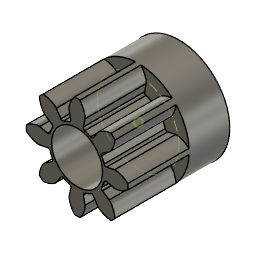
Spur_Gear_Pot (Autodesk Fusion 360 design; units mm, degrees)
description: Spur Gear; Diametrial Pitch: 20.0; Num Teeth: 8; Pressure Angle: 20.0; Backlash: 0.00 in
Autodesk Fusion 360 part; units mm, degrees
(part 1 of 2)
sketch "Sketch1" plane through (0, 0, 7.62) normal (0, 0, 1) x (1, 0, 0)
  arc A0 (5.8346, -2.5905) -> (6.243, -1.3337) centre (0, 0) ccw
  arc A1 (6.5346, -1.1365) -> (6.243, -1.3337) centre (6.4914, -1.3868) ccw
  line L0 (6.5346, -1.1365) -> (7.8387, -1.3616)
  spline S0 degree 5 poles (7.8387, -1.3616) (7.8451, -1.3627) (7.8581, -1.3647) (7.8776, -1.3671) (7.9036, -1.3689) (7.9364, -1.3696) (7.9694, -1.369) (8.0024, -1.3676) (8.0355, -1.3658) (8.0687, -1.3637) (8.1019, -1.3613) (8.1351, -1.3585) (8.1684, -1.3551) (8.2017, -1.3512) (8.235, -1.3466) (8.2684, -1.3414) (8.3019, -1.3357) (8.3353, -1.3297) (8.3688, -1.3232) (8.4023, -1.3164) (8.4358, -1.3093) (8.4693, -1.3017) (8.5028, -1.2938) (8.5363, -1.2855) (8.5698, -1.2768) (8.6034, -1.2677) (8.6369, -1.2583) (8.6704, -1.2484) (8.7039, -1.2383) (8.7374, -1.2278) (8.7709, -1.217) (8.8044, -1.2059) (8.8379, -1.1944) (8.8714, -1.1827) (8.9048, -1.1705) (8.9382, -1.1581) (8.9716, -1.1454) (9.005, -1.1323) (9.0384, -1.1189) (9.0717, -1.1053) (9.105, -1.0913) (9.1383, -1.077) (9.1716, -1.0625) (9.2048, -1.0476) (9.238, -1.0324) (9.2711, -1.017) (9.3042, -1.0013) (9.3373, -0.9852) (9.3703, -0.9689) (9.4033, -0.9524) (9.4363, -0.9355) (9.4692, -0.9184) (9.502, -0.901) (9.5349, -0.8833) (9.5676, -0.8653) (9.6003, -0.8471) (9.633, -0.8286) (9.6656, -0.8098) (9.6982, -0.7908) (9.7307, -0.7715) (9.7632, -0.752) (9.7956, -0.7322) (9.8279, -0.7121) (9.8602, -0.6918) (9.8924, -0.6712) (9.9246, -0.6503) (9.9567, -0.6292) (9.9887, -0.6079) (10.0207, -0.5863) (10.0525, -0.5645) (10.0844, -0.5424) (10.1098, -0.5245) (10.1288, -0.511) (10.1415, -0.5019) (10.1478, -0.4974) knots 0 0 0 0 0 0 0.01428571 0.02857143 0.04285714 0.05714286 0.07142857 0.08571429 0.1 0.11428571 0.12857143 0.14285714 0.15714286 0.17142857 0.18571429 0.2 0.21428571 0.22857143 0.24285714 0.25714286 0.27142857 0.28571429 0.3 0.31428571 0.32857143 0.34285714 0.35714286 0.37142857 0.38571429 0.4 0.41428571 0.42857143 0.44285714 0.45714286 0.47142857 0.48571429 0.5 0.51428571 0.52857143 0.54285714 0.55714286 0.57142857 0.58571429 0.6 0.61428571 0.62857143 0.64285714 0.65714286 0.67142857 0.68571429 0.7 0.71428571 0.72857143 0.74285714 0.75714286 0.77142857 0.78571429 0.8 0.81428571 0.82857143 0.84285714 0.85714286 0.87142857 0.88571429 0.9 0.91428571 0.92857143 0.94285714 0.95714286 0.97142857 0.98571429 1 1 1 1 1 1
  arc A2 (10.1478, -0.4974) -> (10.1478, 0.4974) centre (0, 0) ccw
  spline S1 degree 5 poles (10.1478, 0.4974) (10.1415, 0.5019) (10.1288, 0.511) (10.1098, 0.5245) (10.0844, 0.5424) (10.0525, 0.5645) (10.0207, 0.5863) (9.9887, 0.6079) (9.9567, 0.6292) (9.9246, 0.6503) (9.8924, 0.6712) (9.8602, 0.6918) (9.8279, 0.7121) (9.7956, 0.7322) (9.7632, 0.752) (9.7307, 0.7715) (9.6982, 0.7908) (9.6656, 0.8098) (9.633, 0.8286) (9.6003, 0.8471) (9.5676, 0.8653) (9.5349, 0.8833) (9.502, 0.901) (9.4692, 0.9184) (9.4363, 0.9355) (9.4033, 0.9524) (9.3703, 0.9689) (9.3373, 0.9852) (9.3042, 1.0013) (9.2711, 1.017) (9.238, 1.0324) (9.2048, 1.0476) (9.1716, 1.0625) (9.1383, 1.077) (9.105, 1.0913) (9.0717, 1.1053) (9.0384, 1.1189) (9.005, 1.1323) (8.9716, 1.1454) (8.9382, 1.1581) (8.9048, 1.1705) (8.8714, 1.1827) (8.8379, 1.1944) (8.8044, 1.2059) (8.7709, 1.217) (8.7374, 1.2278) (8.7039, 1.2383) (8.6704, 1.2484) (8.6369, 1.2583) (8.6034, 1.2677) (8.5698, 1.2768) (8.5363, 1.2855) (8.5028, 1.2938) (8.4693, 1.3017) (8.4358, 1.3093) (8.4023, 1.3164) (8.3688, 1.3232) (8.3353, 1.3297) (8.3019, 1.3357) (8.2684, 1.3414) (8.235, 1.3466) (8.2017, 1.3512) (8.1684, 1.3551) (8.1351, 1.3585) (8.1019, 1.3613) (8.0687, 1.3637) (8.0355, 1.3658) (8.0024, 1.3676) (7.9694, 1.369) (7.9364, 1.3696) (7.9036, 1.3689) (7.8776, 1.3671) (7.8581, 1.3647) (7.8451, 1.3627) (7.8387, 1.3616) knots -1 -1 -1 -1 -1 -1 -0.98571429 -0.97142857 -0.95714286 -0.94285714 -0.92857143 -0.91428571 -0.9 -0.88571429 -0.87142857 -0.85714286 -0.84285714 -0.82857143 -0.81428571 -0.8 -0.78571429 -0.77142857 -0.75714286 -0.74285714 -0.72857143 -0.71428571 -0.7 -0.68571429 -0.67142857 -0.65714286 -0.64285714 -0.62857143 -0.61428571 -0.6 -0.58571429 -0.57142857 -0.55714286 -0.54285714 -0.52857143 -0.51428571 -0.5 -0.48571429 -0.47142857 -0.45714286 -0.44285714 -0.42857143 -0.41428571 -0.4 -0.38571429 -0.37142857 -0.35714286 -0.34285714 -0.32857143 -0.31428571 -0.3 -0.28571429 -0.27142857 -0.25714286 -0.24285714 -0.22857143 -0.21428571 -0.2 -0.18571429 -0.17142857 -0.15714286 -0.14285714 -0.12857143 -0.11428571 -0.1 -0.08571429 -0.07142857 -0.05714286 -0.04285714 -0.02857143 -0.01428571 0 0 0 0 0 0
  line L1 (7.8387, 1.3616) -> (6.5346, 1.1365)
  arc A3 (6.243, 1.3337) -> (6.5346, 1.1365) centre (6.4914, 1.3868) ccw
  arc A4 (6.243, 1.3337) -> (5.8346, 2.5905) centre (0, 0) ccw
  arc A5 (5.9546, 2.9215) -> (5.8346, 2.5905) centre (6.0668, 2.6936) ccw
  line L2 (5.9546, 2.9215) -> (7.142, 3.5059)
  spline S2 degree 5 poles (7.142, 3.5059) (7.1478, 3.5088) (7.1595, 3.5148) (7.1766, 3.5243) (7.1988, 3.5382) (7.2257, 3.5569) (7.252, 3.5768) (7.2779, 3.5973) (7.3037, 3.6182) (7.3293, 3.6394) (7.3547, 3.6608) (7.3799, 3.6826) (7.4049, 3.7049) (7.4295, 3.7277) (7.4538, 3.751) (7.4778, 3.7748) (7.5015, 3.7991) (7.525, 3.8237) (7.5483, 3.8486) (7.5714, 3.8737) (7.5943, 3.8992) (7.6169, 3.925) (7.6394, 3.9511) (7.6616, 3.9775) (7.6836, 4.0043) (7.7054, 4.0313) (7.727, 4.0587) (7.7483, 4.0863) (7.7695, 4.1142) (7.7904, 4.1424) (7.8112, 4.1708) (7.8318, 4.1995) (7.8521, 4.2285) (7.8722, 4.2577) (7.8922, 4.2871) (7.9119, 4.3168) (7.9314, 4.3468) (7.9508, 4.377) (7.9699, 4.4074) (7.9888, 4.4381) (8.0076, 4.4689) (8.0261, 4.5) (8.0444, 4.5314) (8.0626, 4.5629) (8.0805, 4.5947) (8.0983, 4.6266) (8.1158, 4.6588) (8.1331, 4.6912) (8.1503, 4.7238) (8.1672, 4.7566) (8.184, 4.7897) (8.2005, 4.8229) (8.2169, 4.8563) (8.233, 4.8899) (8.249, 4.9236) (8.2648, 4.9576) (8.2803, 4.9918) (8.2957, 5.0261) (8.3108, 5.0607) (8.3258, 5.0954) (8.3406, 5.1303) (8.3551, 5.1654) (8.3695, 5.2006) (8.3837, 5.236) (8.3976, 5.2716) (8.4114, 5.3074) (8.425, 5.3433) (8.4383, 5.3794) (8.4515, 5.4157) (8.4645, 5.4521) (8.4772, 5.4887) (8.4873, 5.518) (8.4947, 5.5402) (8.4997, 5.5549) (8.5021, 5.5623) knots 0 0 0 0 0 0 0.01428571 0.02857143 0.04285714 0.05714286 0.07142857 0.08571429 0.1 0.11428571 0.12857143 0.14285714 0.15714286 0.17142857 0.18571429 0.2 0.21428571 0.22857143 0.24285714 0.25714286 0.27142857 0.28571429 0.3 0.31428571 0.32857143 0.34285714 0.35714286 0.37142857 0.38571429 0.4 0.41428571 0.42857143 0.44285714 0.45714286 0.47142857 0.48571429 0.5 0.51428571 0.52857143 0.54285714 0.55714286 0.57142857 0.58571429 0.6 0.61428571 0.62857143 0.64285714 0.65714286 0.67142857 0.68571429 0.7 0.71428571 0.72857143 0.74285714 0.75714286 0.77142857 0.78571429 0.8 0.81428571 0.82857143 0.84285714 0.85714286 0.87142857 0.88571429 0.9 0.91428571 0.92857143 0.94285714 0.95714286 0.97142857 0.98571429 1 1 1 1 1 1
  arc A6 (8.5021, 5.5623) -> (7.9174, 6.3671) centre (0, 0) ccw
  spline S3 degree 5 poles (7.9174, 6.3671) (7.9096, 6.3671) (7.894, 6.367) (7.8707, 6.3667) (7.8396, 6.3662) (7.8009, 6.3654) (7.7623, 6.3643) (7.7237, 6.363) (7.6852, 6.3615) (7.6469, 6.3596) (7.6086, 6.3576) (7.5705, 6.3553) (7.5324, 6.3528) (7.4944, 6.35) (7.4566, 6.347) (7.4188, 6.3437) (7.3812, 6.3402) (7.3437, 6.3365) (7.3062, 6.3325) (7.2689, 6.3283) (7.2317, 6.3238) (7.1947, 6.319) (7.1577, 6.314) (7.1209, 6.3088) (7.0842, 6.3033) (7.0477, 6.2976) (7.0112, 6.2916) (6.9749, 6.2854) (6.9387, 6.2789) (6.9027, 6.2722) (6.8668, 6.2652) (6.8311, 6.2579) (6.7954, 6.2504) (6.76, 6.2427) (6.7247, 6.2347) (6.6895, 6.2264) (6.6545, 6.2179) (6.6197, 6.2091) (6.585, 6.2) (6.5505, 6.1907) (6.5161, 6.1811) (6.4819, 6.1713) (6.4479, 6.1611) (6.4141, 6.1507) (6.3805, 6.14) (6.347, 6.1291) (6.3138, 6.1179) (6.2807, 6.1064) (6.2478, 6.0946) (6.2151, 6.0825) (6.1827, 6.0702) (6.1504, 6.0575) (6.1184, 6.0445) (6.0866, 6.0313) (6.0551, 6.0176) (6.0238, 6.0037) (5.9927, 5.9896) (5.9619, 5.9751) (5.9312, 5.9604) (5.9009, 5.9453) (5.8708, 5.9298) (5.8411, 5.9139) (5.8118, 5.8976) (5.7829, 5.8807) (5.7544, 5.8635) (5.7261, 5.8459) (5.6981, 5.8281) (5.6702, 5.8101) (5.6427, 5.7918) (5.6157, 5.7729) (5.5895, 5.7531) (5.5695, 5.7363) (5.5552, 5.7229) (5.5459, 5.7137) (5.5413, 5.709) knots -1 -1 -1 -1 -1 -1 -0.98571429 -0.97142857 -0.95714286 -0.94285714 -0.92857143 -0.91428571 -0.9 -0.88571429 -0.87142857 -0.85714286 -0.84285714 -0.82857143 -0.81428571 -0.8 -0.78571429 -0.77142857 -0.75714286 -0.74285714 -0.72857143 -0.71428571 -0.7 -0.68571429 -0.67142857 -0.65714286 -0.64285714 -0.62857143 -0.61428571 -0.6 -0.58571429 -0.57142857 -0.55714286 -0.54285714 -0.52857143 -0.51428571 -0.5 -0.48571429 -0.47142857 -0.45714286 -0.44285714 -0.42857143 -0.41428571 -0.4 -0.38571429 -0.37142857 -0.35714286 -0.34285714 -0.32857143 -0.31428571 -0.3 -0.28571429 -0.27142857 -0.25714286 -0.24285714 -0.22857143 -0.21428571 -0.2 -0.18571429 -0.17142857 -0.15714286 -0.14285714 -0.12857143 -0.11428571 -0.1 -0.08571429 -0.07142857 -0.05714286 -0.04285714 -0.02857143 -0.01428571 0 0 0 0 0 0
  line L3 (5.5413, 5.709) -> (4.6186, 4.7604)
  arc A7 (4.2667, 4.7485) -> (4.6186, 4.7604) centre (4.4365, 4.9375) ccw
  arc A8 (4.2667, 4.7485) -> (3.1976, 5.5253) centre (0, 0) ccw
  arc A9 (3.1002, 5.8636) -> (3.1976, 5.5253) centre (3.3249, 5.7451) ccw
  line L4 (3.1002, 5.8636) -> (3.7172, 7.0343)
  spline S4 degree 5 poles (3.7172, 7.0343) (3.7203, 7.0401) (3.7262, 7.0518) (3.7344, 7.0696) (3.7443, 7.0938) (3.755, 7.1248) (3.7646, 7.1563) (3.7735, 7.1881) (3.7821, 7.2202) (3.7903, 7.2524) (3.7983, 7.2847) (3.8059, 7.3171) (3.813, 7.3498) (3.8195, 7.3827) (3.8254, 7.4159) (3.8308, 7.4492) (3.8358, 7.4828) (3.8403, 7.5165) (3.8446, 7.5503) (3.8484, 7.5843) (3.852, 7.6183) (3.8552, 7.6525) (3.858, 7.6868) (3.8605, 7.7213) (3.8625, 7.7558) (3.8643, 7.7905) (3.8656, 7.8254) (3.8667, 7.8603) (3.8674, 7.8953) (3.8678, 7.9304) (3.8678, 7.9656) (3.8676, 8.0009) (3.8671, 8.0362) (3.8662, 8.0717) (3.865, 8.1073) (3.8635, 8.1429) (3.8617, 8.1786) (3.8596, 8.2144) (3.8572, 8.2502) (3.8545, 8.2862) (3.8515, 8.3222) (3.8482, 8.3582) (3.8446, 8.3943) (3.8407, 8.4305) (3.8366, 8.4668) (3.8321, 8.5031) (3.8274, 8.5394) (3.8224, 8.5758) (3.8171, 8.6123) (3.8115, 8.6488) (3.8057, 8.6853) (3.7996, 8.7219) (3.7932, 8.7586) (3.7865, 8.7952) (3.7795, 8.832) (3.7723, 8.8687) (3.7648, 8.9055) (3.757, 8.9423) (3.749, 8.9792) (3.7407, 9.016) (3.7322, 9.0529) (3.7233, 9.0899) (3.7142, 9.1268) (3.7049, 9.1638) (3.6953, 9.2008) (3.6854, 9.2379) (3.6752, 9.2749) (3.6648, 9.312) (3.6542, 9.349) (3.6433, 9.3861) (3.6321, 9.4232) (3.6229, 9.4529) (3.616, 9.4752) (3.6113, 9.49) (3.6089, 9.4974) knots 0 0 0 0 0 0 0.01428571 0.02857143 0.04285714 0.05714286 0.07142857 0.08571429 0.1 0.11428571 0.12857143 0.14285714 0.15714286 0.17142857 0.18571429 0.2 0.21428571 0.22857143 0.24285714 0.25714286 0.27142857 0.28571429 0.3 0.31428571 0.32857143 0.34285714 0.35714286 0.37142857 0.38571429 0.4 0.41428571 0.42857143 0.44285714 0.45714286 0.47142857 0.48571429 0.5 0.51428571 0.52857143 0.54285714 0.55714286 0.57142857 0.58571429 0.6 0.61428571 0.62857143 0.64285714 0.65714286 0.67142857 0.68571429 0.7 0.71428571 0.72857143 0.74285714 0.75714286 0.77142857 0.78571429 0.8 0.81428571 0.82857143 0.84285714 0.85714286 0.87142857 0.88571429 0.9 0.91428571 0.92857143 0.94285714 0.95714286 0.97142857 0.98571429 1 1 1 1 1 1
  arc A10 (3.6089, 9.4974) -> (2.6628, 9.8049) centre (0, 0) ccw
  spline S5 degree 5 poles (2.6628, 9.8049) (2.6565, 9.8002) (2.644, 9.791) (2.6253, 9.7771) (2.6004, 9.7584) (2.5696, 9.735) (2.5389, 9.7114) (2.5085, 9.6877) (2.4783, 9.6638) (2.4483, 9.6398) (2.4186, 9.6156) (2.3891, 9.5914) (2.3598, 9.5669) (2.3307, 9.5424) (2.3018, 9.5177) (2.2732, 9.4929) (2.2448, 9.4679) (2.2166, 9.4428) (2.1887, 9.4176) (2.161, 9.3922) (2.1336, 9.3667) (2.1064, 9.3411) (2.0794, 9.3154) (2.0527, 9.2895) (2.0262, 9.2635) (2, 9.2374) (1.9741, 9.2111) (1.9484, 9.1847) (1.9229, 9.1582) (1.8977, 9.1316) (1.8728, 9.1049) (1.8481, 9.078) (1.8237, 9.051) (1.7996, 9.0239) (1.7757, 8.9966) (1.7522, 8.9693) (1.7289, 8.9418) (1.7058, 8.9142) (1.6831, 8.8865) (1.6606, 8.8586) (1.6385, 8.8307) (1.6166, 8.8026) (1.5951, 8.7745) (1.5738, 8.7462) (1.5529, 8.7178) (1.5323, 8.6892) (1.512, 8.6606) (1.492, 8.6319) (1.4723, 8.603) (1.4529, 8.574) (1.4339, 8.545) (1.4153, 8.5158) (1.397, 8.4865) (1.3791, 8.457) (1.3616, 8.4275) (1.3445, 8.3978) (1.3276, 8.3681) (1.3112, 8.3383) (1.2951, 8.3083) (1.2793, 8.2783) (1.2641, 8.2481) (1.2494, 8.2178) (1.2353, 8.1873) (1.2219, 8.1567) (1.2089, 8.126) (1.1964, 8.0952) (1.1842, 8.0643) (1.1722, 8.0334) (1.1607, 8.0024) (1.15, 7.9712) (1.1404, 7.9398) (1.1342, 7.9144) (1.1304, 7.8952) (1.1283, 7.8823) (1.1273, 7.8758) knots -1 -1 -1 -1 -1 -1 -0.98571429 -0.97142857 -0.95714286 -0.94285714 -0.92857143 -0.91428571 -0.9 -0.88571429 -0.87142857 -0.85714286 -0.84285714 -0.82857143 -0.81428571 -0.8 -0.78571429 -0.77142857 -0.75714286 -0.74285714 -0.72857143 -0.71428571 -0.7 -0.68571429 -0.67142857 -0.65714286 -0.64285714 -0.62857143 -0.61428571 -0.6 -0.58571429 -0.57142857 -0.55714286 -0.54285714 -0.52857143 -0.51428571 -0.5 -0.48571429 -0.47142857 -0.45714286 -0.44285714 -0.42857143 -0.41428571 -0.4 -0.38571429 -0.37142857 -0.35714286 -0.34285714 -0.32857143 -0.31428571 -0.3 -0.28571429 -0.27142857 -0.25714286 -0.24285714 -0.22857143 -0.21428571 -0.2 -0.18571429 -0.17142857 -0.15714286 -0.14285714 -0.12857143 -0.11428571 -0.1 -0.08571429 -0.07142857 -0.05714286 -0.04285714 -0.02857143 -0.01428571 0 0 0 0 0 0
  line L5 (1.1273, 7.8758) -> (0.9384, 6.566)
  arc A11 (0.6607, 6.3496) -> (0.9384, 6.566) centre (0.687, 6.6022) ccw
  arc A12 (0.6607, 6.3496) -> (-0.6607, 6.3496) centre (0, 0) ccw
  arc A13 (-0.9384, 6.566) -> (-0.6607, 6.3496) centre (-0.687, 6.6022) ccw
  line L6 (-0.9384, 6.566) -> (-1.1273, 7.8758)
  spline S6 degree 5 poles (-1.1273, 7.8758) (-1.1283, 7.8823) (-1.1304, 7.8952) (-1.1342, 7.9144) (-1.1404, 7.9398) (-1.15, 7.9712) (-1.1607, 8.0024) (-1.1722, 8.0334) (-1.1842, 8.0643) (-1.1964, 8.0952) (-1.2089, 8.126) (-1.2219, 8.1567) (-1.2353, 8.1873) (-1.2494, 8.2178) (-1.2641, 8.2481) (-1.2793, 8.2783) (-1.2951, 8.3083) (-1.3112, 8.3383) (-1.3276, 8.3681) (-1.3445, 8.3978) (-1.3616, 8.4275) (-1.3791, 8.457) (-1.397, 8.4865) (-1.4153, 8.5158) (-1.4339, 8.545) (-1.4529, 8.574) (-1.4723, 8.603) (-1.492, 8.6319) (-1.512, 8.6606) (-1.5323, 8.6892) (-1.5529, 8.7178) (-1.5738, 8.7462) (-1.5951, 8.7745) (-1.6166, 8.8026) (-1.6385, 8.8307) (-1.6606, 8.8586) (-1.6831, 8.8865) (-1.7058, 8.9142) (-1.7289, 8.9418) (-1.7522, 8.9693) (-1.7757, 8.9966) (-1.7996, 9.0239) (-1.8237, 9.051) (-1.8481, 9.078) (-1.8728, 9.1049) (-1.8977, 9.1316) (-1.9229, 9.1582) (-1.9484, 9.1847) (-1.9741, 9.2111) (-2, 9.2374) (-2.0262, 9.2635) (-2.0527, 9.2895) (-2.0794, 9.3154) (-2.1064, 9.3411) (-2.1336, 9.3667) (-2.161, 9.3922) (-2.1887, 9.4176) (-2.2166, 9.4428) (-2.2448, 9.4679) (-2.2732, 9.4929) (-2.3018, 9.5177) (-2.3307, 9.5424) (-2.3598, 9.5669) (-2.3891, 9.5914) (-2.4186, 9.6156) (-2.4483, 9.6398) (-2.4783, 9.6638) (-2.5085, 9.6877) (-2.5389, 9.7114) (-2.5696, 9.735) (-2.6004, 9.7584) (-2.6253, 9.7771) (-2.644, 9.791) (-2.6565, 9.8002) (-2.6628, 9.8049) knots 0 0 0 0 0 0 0.01428571 0.02857143 0.04285714 0.05714286 0.07142857 0.08571429 0.1 0.11428571 0.12857143 0.14285714 0.15714286 0.17142857 0.18571429 0.2 0.21428571 0.22857143 0.24285714 0.25714286 0.27142857 0.28571429 0.3 0.31428571 0.32857143 0.34285714 0.35714286 0.37142857 0.38571429 0.4 0.41428571 0.42857143 0.44285714 0.45714286 0.47142857 0.48571429 0.5 0.51428571 0.52857143 0.54285714 0.55714286 0.57142857 0.58571429 0.6 0.61428571 0.62857143 0.64285714 0.65714286 0.67142857 0.68571429 0.7 0.71428571 0.72857143 0.74285714 0.75714286 0.77142857 0.78571429 0.8 0.81428571 0.82857143 0.84285714 0.85714286 0.87142857 0.88571429 0.9 0.91428571 0.92857143 0.94285714 0.95714286 0.97142857 0.98571429 1 1 1 1 1 1
  arc A14 (-2.6628, 9.8049) -> (-3.6089, 9.4974) centre (0, 0) ccw
  spline S7 degree 5 poles (-3.6089, 9.4974) (-3.6113, 9.49) (-3.616, 9.4752) (-3.6229, 9.4529) (-3.6321, 9.4232) (-3.6433, 9.3861) (-3.6542, 9.349) (-3.6648, 9.312) (-3.6752, 9.2749) (-3.6854, 9.2379) (-3.6953, 9.2008) (-3.7049, 9.1638) (-3.7142, 9.1268) (-3.7233, 9.0899) (-3.7322, 9.0529) (-3.7407, 9.016) (-3.749, 8.9792) (-3.757, 8.9423) (-3.7648, 8.9055) (-3.7723, 8.8687) (-3.7795, 8.832) (-3.7865, 8.7952) (-3.7932, 8.7586) (-3.7996, 8.7219) (-3.8057, 8.6853) (-3.8115, 8.6488) (-3.8171, 8.6123) (-3.8224, 8.5758) (-3.8274, 8.5394) (-3.8321, 8.5031) (-3.8366, 8.4668) (-3.8407, 8.4305) (-3.8446, 8.3943) (-3.8482, 8.3582) (-3.8515, 8.3222) (-3.8545, 8.2862) (-3.8572, 8.2502) (-3.8596, 8.2144) (-3.8617, 8.1786) (-3.8635, 8.1429) (-3.865, 8.1073) (-3.8662, 8.0717) (-3.8671, 8.0362) (-3.8676, 8.0009) (-3.8678, 7.9656) (-3.8678, 7.9304) (-3.8674, 7.8953) (-3.8667, 7.8603) (-3.8656, 7.8254) (-3.8643, 7.7905) (-3.8625, 7.7558) (-3.8605, 7.7213) (-3.858, 7.6868) (-3.8552, 7.6525) (-3.852, 7.6183) (-3.8484, 7.5843) (-3.8446, 7.5503) (-3.8403, 7.5165) (-3.8358, 7.4828) (-3.8308, 7.4492) (-3.8254, 7.4159) (-3.8195, 7.3827) (-3.813, 7.3498) (-3.8059, 7.3171) (-3.7983, 7.2847) (-3.7903, 7.2524) (-3.7821, 7.2202) (-3.7735, 7.1881) (-3.7646, 7.1563) (-3.755, 7.1248) (-3.7443, 7.0938) (-3.7344, 7.0696) (-3.7262, 7.0518) (-3.7203, 7.0401) (-3.7172, 7.0343) knots -1 -1 -1 -1 -1 -1 -0.98571429 -0.97142857 -0.95714286 -0.94285714 -0.92857143 -0.91428571 -0.9 -0.88571429 -0.87142857 -0.85714286 -0.84285714 -0.82857143 -0.81428571 -0.8 -0.78571429 -0.77142857 -0.75714286 -0.74285714 -0.72857143 -0.71428571 -0.7 -0.68571429 -0.67142857 -0.65714286 -0.64285714 -0.62857143 -0.61428571 -0.6 -0.58571429 -0.57142857 -0.55714286 -0.54285714 -0.52857143 -0.51428571 -0.5 -0.48571429 -0.47142857 -0.45714286 -0.44285714 -0.42857143 -0.41428571 -0.4 -0.38571429 -0.37142857 -0.35714286 -0.34285714 -0.32857143 -0.31428571 -0.3 -0.28571429 -0.27142857 -0.25714286 -0.24285714 -0.22857143 -0.21428571 -0.2 -0.18571429 -0.17142857 -0.15714286 -0.14285714 -0.12857143 -0.11428571 -0.1 -0.08571429 -0.07142857 -0.05714286 -0.04285714 -0.02857143 -0.01428571 0 0 0 0 0 0
  line L7 (-3.7172, 7.0343) -> (-3.1002, 5.8636)
  arc A15 (-3.1976, 5.5253) -> (-3.1002, 5.8636) centre (-3.3249, 5.7451) ccw
  arc A16 (-3.1976, 5.5253) -> (-4.2667, 4.7485) centre (0, 0) ccw
  arc A17 (-4.6186, 4.7604) -> (-4.2667, 4.7485) centre (-4.4365, 4.9375) ccw
  line L8 (-4.6186, 4.7604) -> (-5.5413, 5.709)
  spline S8 degree 5 poles (-5.5413, 5.709) (-5.5459, 5.7137) (-5.5552, 5.7229) (-5.5695, 5.7363) (-5.5895, 5.7531) (-5.6157, 5.7729) (-5.6427, 5.7918) (-5.6702, 5.8101) (-5.6981, 5.8281) (-5.7261, 5.8459) (-5.7544, 5.8635) (-5.7829, 5.8807) (-5.8118, 5.8976) (-5.8411, 5.9139) (-5.8708, 5.9298) (-5.9009, 5.9453) (-5.9312, 5.9604) (-5.9619, 5.9751) (-5.9927, 5.9896) (-6.0238, 6.0037) (-6.0551, 6.0176) (-6.0866, 6.0313) (-6.1184, 6.0445) (-6.1504, 6.0575) (-6.1827, 6.0702) (-6.2151, 6.0825) (-6.2478, 6.0946) (-6.2807, 6.1064) (-6.3138, 6.1179) (-6.347, 6.1291) (-6.3805, 6.14) (-6.4141, 6.1507) (-6.4479, 6.1611) (-6.4819, 6.1713) (-6.5161, 6.1811) (-6.5505, 6.1907) (-6.585, 6.2) (-6.6197, 6.2091) (-6.6545, 6.2179) (-6.6895, 6.2264) (-6.7247, 6.2347) (-6.76, 6.2427) (-6.7954, 6.2504) (-6.8311, 6.2579) (-6.8668, 6.2652) (-6.9027, 6.2722) (-6.9387, 6.2789) (-6.9749, 6.2854) (-7.0112, 6.2916) (-7.0477, 6.2976) (-7.0842, 6.3033) (-7.1209, 6.3088) (-7.1577, 6.314) (-7.1947, 6.319) (-7.2317, 6.3238) (-7.2689, 6.3283) (-7.3062, 6.3325) (-7.3437, 6.3365) (-7.3812, 6.3402) (-7.4188, 6.3437) (-7.4566, 6.347) (-7.4944, 6.35) (-7.5324, 6.3528) (-7.5705, 6.3553) (-7.6086, 6.3576) (-7.6469, 6.3596) (-7.6852, 6.3615) (-7.7237, 6.363) (-7.7623, 6.3643) (-7.8009, 6.3654) (-7.8396, 6.3662) (-7.8707, 6.3667) (-7.894, 6.367) (-7.9096, 6.3671) (-7.9174, 6.3671) knots 0 0 0 0 0 0 0.01428571 0.02857143 0.04285714 0.05714286 0.07142857 0.08571429 0.1 0.11428571 0.12857143 0.14285714 0.15714286 0.17142857 0.18571429 0.2 0.21428571 0.22857143 0.24285714 0.25714286 0.27142857 0.28571429 0.3 0.31428571 0.32857143 0.34285714 0.35714286 0.37142857 0.38571429 0.4 0.41428571 0.42857143 0.44285714 0.45714286 0.47142857 0.48571429 0.5 0.51428571 0.52857143 0.54285714 0.55714286 0.57142857 0.58571429 0.6 0.61428571 0.62857143 0.64285714 0.65714286 0.67142857 0.68571429 0.7 0.71428571 0.72857143 0.74285714 0.75714286 0.77142857 0.78571429 0.8 0.81428571 0.82857143 0.84285714 0.85714286 0.87142857 0.88571429 0.9 0.91428571 0.92857143 0.94285714 0.95714286 0.97142857 0.98571429 1 1 1 1 1 1
  arc A18 (-7.9174, 6.3671) -> (-8.5021, 5.5623) centre (0, 0) ccw
  spline S9 degree 5 poles (-8.5021, 5.5623) (-8.4997, 5.5549) (-8.4947, 5.5402) (-8.4873, 5.518) (-8.4772, 5.4887) (-8.4645, 5.4521) (-8.4515, 5.4157) (-8.4383, 5.3794) (-8.425, 5.3433) (-8.4114, 5.3074) (-8.3976, 5.2716) (-8.3837, 5.236) (-8.3695, 5.2006) (-8.3551, 5.1654) (-8.3406, 5.1303) (-8.3258, 5.0954) (-8.3108, 5.0607) (-8.2957, 5.0261) (-8.2803, 4.9918) (-8.2648, 4.9576) (-8.249, 4.9236) (-8.233, 4.8899) (-8.2169, 4.8563) (-8.2005, 4.8229) (-8.184, 4.7897) (-8.1672, 4.7566) (-8.1503, 4.7238) (-8.1331, 4.6912) (-8.1158, 4.6588) (-8.0983, 4.6266) (-8.0805, 4.5947) (-8.0626, 4.5629) (-8.0444, 4.5314) (-8.0261, 4.5) (-8.0076, 4.4689) (-7.9888, 4.4381) (-7.9699, 4.4074) (-7.9508, 4.377) (-7.9314, 4.3468) (-7.9119, 4.3168) (-7.8922, 4.2871) (-7.8722, 4.2577) (-7.8521, 4.2285) (-7.8318, 4.1995) (-7.8112, 4.1708) (-7.7904, 4.1424) (-7.7695, 4.1142) (-7.7483, 4.0863) (-7.727, 4.0587) (-7.7054, 4.0313) (-7.6836, 4.0043) (-7.6616, 3.9775) (-7.6394, 3.9511) (-7.6169, 3.925) (-7.5943, 3.8992) (-7.5714, 3.8737) (-7.5483, 3.8486) (-7.525, 3.8237) (-7.5015, 3.7991) (-7.4778, 3.7748) (-7.4538, 3.751) (-7.4295, 3.7277) (-7.4049, 3.7049) (-7.3799, 3.6826) (-7.3547, 3.6608) (-7.3293, 3.6394) (-7.3037, 3.6182) (-7.2779, 3.5973) (-7.252, 3.5768) (-7.2257, 3.5569) (-7.1988, 3.5382) (-7.1766, 3.5243) (-7.1595, 3.5148) (-7.1478, 3.5088) (-7.142, 3.5059) knots -1 -1 -1 -1 -1 -1 -0.98571429 -0.97142857 -0.95714286 -0.94285714 -0.92857143 -0.91428571 -0.9 -0.88571429 -0.87142857 -0.85714286 -0.84285714 -0.82857143 -0.81428571 -0.8 -0.78571429 -0.77142857 -0.75714286 -0.74285714 -0.72857143 -0.71428571 -0.7 -0.68571429 -0.67142857 -0.65714286 -0.64285714 -0.62857143 -0.61428571 -0.6 -0.58571429 -0.57142857 -0.55714286 -0.54285714 -0.52857143 -0.51428571 -0.5 -0.48571429 -0.47142857 -0.45714286 -0.44285714 -0.42857143 -0.41428571 -0.4 -0.38571429 -0.37142857 -0.35714286 -0.34285714 -0.32857143 -0.31428571 -0.3 -0.28571429 -0.27142857 -0.25714286 -0.24285714 -0.22857143 -0.21428571 -0.2 -0.18571429 -0.17142857 -0.15714286 -0.14285714 -0.12857143 -0.11428571 -0.1 -0.08571429 -0.07142857 -0.05714286 -0.04285714 -0.02857143 -0.01428571 0 0 0 0 0 0
  line L9 (-7.142, 3.5059) -> (-5.9546, 2.9215)
  arc A19 (-5.8346, 2.5905) -> (-5.9546, 2.9215) centre (-6.0668, 2.6936) ccw
  arc A20 (-5.8346, 2.5905) -> (-6.243, 1.3337) centre (0, 0) ccw
  arc A21 (-6.5346, 1.1365) -> (-6.243, 1.3337) centre (-6.4914, 1.3868) ccw
  line L10 (-6.5346, 1.1365) -> (-7.8387, 1.3616)
  spline S10 degree 5 poles (-7.8387, 1.3616) (-7.8451, 1.3627) (-7.8581, 1.3647) (-7.8776, 1.3671) (-7.9036, 1.3689) (-7.9364, 1.3696) (-7.9694, 1.369) (-8.0024, 1.3676) (-8.0355, 1.3658) (-8.0687, 1.3637) (-8.1019, 1.3613) (-8.1351, 1.3585) (-8.1684, 1.3551) (-8.2017, 1.3512) (-8.235, 1.3466) (-8.2684, 1.3414) (-8.3019, 1.3357) (-8.3353, 1.3297) (-8.3688, 1.3232) (-8.4023, 1.3164) (-8.4358, 1.3093) (-8.4693, 1.3017) (-8.5028, 1.2938) (-8.5363, 1.2855) (-8.5698, 1.2768) (-8.6034, 1.2677) (-8.6369, 1.2583) (-8.6704, 1.2484) (-8.7039, 1.2383) (-8.7374, 1.2278) (-8.7709, 1.217) (-8.8044, 1.2059) (-8.8379, 1.1944) (-8.8714, 1.1827) (-8.9048, 1.1705) (-8.9382, 1.1581) (-8.9716, 1.1454) (-9.005, 1.1323) (-9.0384, 1.1189) (-9.0717, 1.1053) (-9.105, 1.0913) (-9.1383, 1.077) (-9.1716, 1.0625) (-9.2048, 1.0476) (-9.238, 1.0324) (-9.2711, 1.017) (-9.3042, 1.0013) (-9.3373, 0.9852) (-9.3703, 0.9689) (-9.4033, 0.9524) (-9.4363, 0.9355) (-9.4692, 0.9184) (-9.502, 0.901) (-9.5349, 0.8833) (-9.5676, 0.8653) (-9.6003, 0.8471) (-9.633, 0.8286) (-9.6656, 0.8098) (-9.6982, 0.7908) (-9.7307, 0.7715) (-9.7632, 0.752) (-9.7956, 0.7322) (-9.8279, 0.7121) (-9.8602, 0.6918) (-9.8924, 0.6712) (-9.9246, 0.6503) (-9.9567, 0.6292) (-9.9887, 0.6079) (-10.0207, 0.5863) (-10.0525, 0.5645) (-10.0844, 0.5424) (-10.1098, 0.5245) (-10.1288, 0.511) (-10.1415, 0.5019) (-10.1478, 0.4974) knots 0 0 0 0 0 0 0.01428571 0.02857143 0.04285714 0.05714286 0.07142857 0.08571429 0.1 0.11428571 0.12857143 0.14285714 0.15714286 0.17142857 0.18571429 0.2 0.21428571 0.22857143 0.24285714 0.25714286 0.27142857 0.28571429 0.3 0.31428571 0.32857143 0.34285714 0.35714286 0.37142857 0.38571429 0.4 0.41428571 0.42857143 0.44285714 0.45714286 0.47142857 0.48571429 0.5 0.51428571 0.52857143 0.54285714 0.55714286 0.57142857 0.58571429 0.6 0.61428571 0.62857143 0.64285714 0.65714286 0.67142857 0.68571429 0.7 0.71428571 0.72857143 0.74285714 0.75714286 0.77142857 0.78571429 0.8 0.81428571 0.82857143 0.84285714 0.85714286 0.87142857 0.88571429 0.9 0.91428571 0.92857143 0.94285714 0.95714286 0.97142857 0.98571429 1 1 1 1 1 1
  arc A22 (-10.1478, 0.4974) -> (-10.1478, -0.4974) centre (0, 0) ccw
  spline S11 degree 5 poles (-10.1478, -0.4974) (-10.1415, -0.5019) (-10.1288, -0.511) (-10.1098, -0.5245) (-10.0844, -0.5424) (-10.0525, -0.5645) (-10.0207, -0.5863) (-9.9887, -0.6079) (-9.9567, -0.6292) (-9.9246, -0.6503) (-9.8924, -0.6712) (-9.8602, -0.6918) (-9.8279, -0.7121) (-9.7956, -0.7322) (-9.7632, -0.752) (-9.7307, -0.7715) (-9.6982, -0.7908) (-9.6656, -0.8098) (-9.633, -0.8286) (-9.6003, -0.8471) (-9.5676, -0.8653) (-9.5349, -0.8833) (-9.502, -0.901) (-9.4692, -0.9184) (-9.4363, -0.9355) (-9.4033, -0.9524) (-9.3703, -0.9689) (-9.3373, -0.9852) (-9.3042, -1.0013) (-9.2711, -1.017) (-9.238, -1.0324) (-9.2048, -1.0476) (-9.1716, -1.0625) (-9.1383, -1.077) (-9.105, -1.0913) (-9.0717, -1.1053) (-9.0384, -1.1189) (-9.005, -1.1323) (-8.9716, -1.1454) (-8.9382, -1.1581) (-8.9048, -1.1705) (-8.8714, -1.1827) (-8.8379, -1.1944) (-8.8044, -1.2059) (-8.7709, -1.217) (-8.7374, -1.2278) (-8.7039, -1.2383) (-8.6704, -1.2484) (-8.6369, -1.2583) (-8.6034, -1.2677) (-8.5698, -1.2768) (-8.5363, -1.2855) (-8.5028, -1.2938) (-8.4693, -1.3017) (-8.4358, -1.3093) (-8.4023, -1.3164) (-8.3688, -1.3232) (-8.3353, -1.3297) (-8.3019, -1.3357) (-8.2684, -1.3414) (-8.235, -1.3466) (-8.2017, -1.3512) (-8.1684, -1.3551) (-8.1351, -1.3585) (-8.1019, -1.3613) (-8.0687, -1.3637) (-8.0355, -1.3658) (-8.0024, -1.3676) (-7.9694, -1.369) (-7.9364, -1.3696) (-7.9036, -1.3689) (-7.8776, -1.3671) (-7.8581, -1.3647) (-7.8451, -1.3627) (-7.8387, -1.3616) knots -1 -1 -1 -1 -1 -1 -0.98571429 -0.97142857 -0.95714286 -0.94285714 -0.92857143 -0.91428571 -0.9 -0.88571429 -0.87142857 -0.85714286 -0.84285714 -0.82857143 -0.81428571 -0.8 -0.78571429 -0.77142857 -0.75714286 -0.74285714 -0.72857143 -0.71428571 -0.7 -0.68571429 -0.67142857 -0.65714286 -0.64285714 -0.62857143 -0.61428571 -0.6 -0.58571429 -0.57142857 -0.55714286 -0.54285714 -0.52857143 -0.51428571 -0.5 -0.48571429 -0.47142857 -0.45714286 -0.44285714 -0.42857143 -0.41428571 -0.4 -0.38571429 -0.37142857 -0.35714286 -0.34285714 -0.32857143 -0.31428571 -0.3 -0.28571429 -0.27142857 -0.25714286 -0.24285714 -0.22857143 -0.21428571 -0.2 -0.18571429 -0.17142857 -0.15714286 -0.14285714 -0.12857143 -0.11428571 -0.1 -0.08571429 -0.07142857 -0.05714286 -0.04285714 -0.02857143 -0.01428571 0 0 0 0 0 0
  line L11 (-7.8387, -1.3616) -> (-6.5346, -1.1365)
  arc A23 (-6.243, -1.3337) -> (-6.5346, -1.1365) centre (-6.4914, -1.3868) ccw
  arc A24 (-6.243, -1.3337) -> (-5.8346, -2.5905) centre (0, 0) ccw
  arc A25 (-5.9546, -2.9215) -> (-5.8346, -2.5905) centre (-6.0668, -2.6936) ccw
  line L12 (-5.9546, -2.9215) -> (-7.142, -3.5059)
  spline S12 degree 5 poles (-7.142, -3.5059) (-7.1478, -3.5088) (-7.1595, -3.5148) (-7.1766, -3.5243) (-7.1988, -3.5382) (-7.2257, -3.5569) (-7.252, -3.5768) (-7.2779, -3.5973) (-7.3037, -3.6182) (-7.3293, -3.6394) (-7.3547, -3.6608) (-7.3799, -3.6826) (-7.4049, -3.7049) (-7.4295, -3.7277) (-7.4538, -3.751) (-7.4778, -3.7748) (-7.5015, -3.7991) (-7.525, -3.8237) (-7.5483, -3.8486) (-7.5714, -3.8737) (-7.5943, -3.8992) (-7.6169, -3.925) (-7.6394, -3.9511) (-7.6616, -3.9775) (-7.6836, -4.0043) (-7.7054, -4.0313) (-7.727, -4.0587) (-7.7483, -4.0863) (-7.7695, -4.1142) (-7.7904, -4.1424) (-7.8112, -4.1708) (-7.8318, -4.1995) (-7.8521, -4.2285) (-7.8722, -4.2577) (-7.8922, -4.2871) (-7.9119, -4.3168) (-7.9314, -4.3468) (-7.9508, -4.377) (-7.9699, -4.4074) (-7.9888, -4.4381) (-8.0076, -4.4689) (-8.0261, -4.5) (-8.0444, -4.5314) (-8.0626, -4.5629) (-8.0805, -4.5947) (-8.0983, -4.6266) (-8.1158, -4.6588) (-8.1331, -4.6912) (-8.1503, -4.7238) (-8.1672, -4.7566) (-8.184, -4.7897) (-8.2005, -4.8229) (-8.2169, -4.8563) (-8.233, -4.8899) (-8.249, -4.9236) (-8.2648, -4.9576) (-8.2803, -4.9918) (-8.2957, -5.0261) (-8.3108, -5.0607) (-8.3258, -5.0954) (-8.3406, -5.1303) (-8.3551, -5.1654) (-8.3695, -5.2006) (-8.3837, -5.236) (-8.3976, -5.2716) (-8.4114, -5.3074) (-8.425, -5.3433) (-8.4383, -5.3794) (-8.4515, -5.4157) (-8.4645, -5.4521) (-8.4772, -5.4887) (-8.4873, -5.518) (-8.4947, -5.5402) (-8.4997, -5.5549) (-8.5021, -5.5623) knots 0 0 0 0 0 0 0.01428571 0.02857143 0.04285714 0.05714286 0.07142857 0.08571429 0.1 0.11428571 0.12857143 0.14285714 0.15714286 0.17142857 0.18571429 0.2 0.21428571 0.22857143 0.24285714 0.25714286 0.27142857 0.28571429 0.3 0.31428571 0.32857143 0.34285714 0.35714286 0.37142857 0.38571429 0.4 0.41428571 0.42857143 0.44285714 0.45714286 0.47142857 0.48571429 0.5 0.51428571 0.52857143 0.54285714 0.55714286 0.57142857 0.58571429 0.6 0.61428571 0.62857143 0.64285714 0.65714286 0.67142857 0.68571429 0.7 0.71428571 0.72857143 0.74285714 0.75714286 0.77142857 0.78571429 0.8 0.81428571 0.82857143 0.84285714 0.85714286 0.87142857 0.88571429 0.9 0.91428571 0.92857143 0.94285714 0.95714286 0.97142857 0.98571429 1 1 1 1 1 1
  arc A26 (-8.5021, -5.5623) -> (-7.9174, -6.3671) centre (0, 0) ccw
  spline S13 degree 5 poles (-7.9174, -6.3671) (-7.9096, -6.3671) (-7.894, -6.367) (-7.8707, -6.3667) (-7.8396, -6.3662) (-7.8009, -6.3654) (-7.7623, -6.3643) (-7.7237, -6.363) (-7.6852, -6.3615) (-7.6469, -6.3596) (-7.6086, -6.3576) (-7.5705, -6.3553) (-7.5324, -6.3528) (-7.4944, -6.35) (-7.4566, -6.347) (-7.4188, -6.3437) (-7.3812, -6.3402) (-7.3437, -6.3365) (-7.3062, -6.3325) (-7.2689, -6.3283) (-7.2317, -6.3238) (-7.1947, -6.319) (-7.1577, -6.314) (-7.1209, -6.3088) (-7.0842, -6.3033) (-7.0477, -6.2976) (-7.0112, -6.2916) (-6.9749, -6.2854) (-6.9387, -6.2789) (-6.9027, -6.2722) (-6.8668, -6.2652) (-6.8311, -6.2579) (-6.7954, -6.2504) (-6.76, -6.2427) (-6.7247, -6.2347) (-6.6895, -6.2264) (-6.6545, -6.2179) (-6.6197, -6.2091) (-6.585, -6.2) (-6.5505, -6.1907) (-6.5161, -6.1811) (-6.4819, -6.1713) (-6.4479, -6.1611) (-6.4141, -6.1507) (-6.3805, -6.14) (-6.347, -6.1291) (-6.3138, -6.1179) (-6.2807, -6.1064) (-6.2478, -6.0946) (-6.2151, -6.0825) (-6.1827, -6.0702) (-6.1504, -6.0575) (-6.1184, -6.0445) (-6.0866, -6.0313) (-6.0551, -6.0176) (-6.0238, -6.0037) (-5.9927, -5.9896) (-5.9619, -5.9751) (-5.9312, -5.9604) (-5.9009, -5.9453) (-5.8708, -5.9298) (-5.8411, -5.9139) (-5.8118, -5.8976) (-5.7829, -5.8807) (-5.7544, -5.8635) (-5.7261, -5.8459) (-5.6981, -5.8281) (-5.6702, -5.8101) (-5.6427, -5.7918) (-5.6157, -5.7729) (-5.5895, -5.7531) (-5.5695, -5.7363) (-5.5552, -5.7229) (-5.5459, -5.7137) (-5.5413, -5.709) knots -1 -1 -1 -1 -1 -1 -0.98571429 -0.97142857 -0.95714286 -0.94285714 -0.92857143 -0.91428571 -0.9 -0.88571429 -0.87142857 -0.85714286 -0.84285714 -0.82857143 -0.81428571 -0.8 -0.78571429 -0.77142857 -0.75714286 -0.74285714 -0.72857143 -0.71428571 -0.7 -0.68571429 -0.67142857 -0.65714286 -0.64285714 -0.62857143 -0.61428571 -0.6 -0.58571429 -0.57142857 -0.55714286 -0.54285714 -0.52857143 -0.51428571 -0.5 -0.48571429 -0.47142857 -0.45714286 -0.44285714 -0.42857143 -0.41428571 -0.4 -0.38571429 -0.37142857 -0.35714286 -0.34285714 -0.32857143 -0.31428571 -0.3 -0.28571429 -0.27142857 -0.25714286 -0.24285714 -0.22857143 -0.21428571 -0.2 -0.18571429 -0.17142857 -0.15714286 -0.14285714 -0.12857143 -0.11428571 -0.1 -0.08571429 -0.07142857 -0.05714286 -0.04285714 -0.02857143 -0.01428571 0 0 0 0 0 0
  line L13 (-5.5413, -5.709) -> (-4.6186, -4.7604)
  arc A27 (-4.2667, -4.7485) -> (-4.6186, -4.7604) centre (-4.4365, -4.9375) ccw
  arc A28 (-4.2667, -4.7485) -> (-3.1976, -5.5253) centre (0, 0) ccw
  arc A29 (-3.1002, -5.8636) -> (-3.1976, -5.5253) centre (-3.3249, -5.7451) ccw
  line L14 (-3.1002, -5.8636) -> (-3.7172, -7.0343)
  spline S14 degree 5 poles (-3.7172, -7.0343) (-3.7203, -7.0401) (-3.7262, -7.0518) (-3.7344, -7.0696) (-3.7443, -7.0938) (-3.755, -7.1248) (-3.7646, -7.1563) (-3.7735, -7.1881) (-3.7821, -7.2202) (-3.7903, -7.2524) (-3.7983, -7.2847) (-3.8059, -7.3171) (-3.813, -7.3498) (-3.8195, -7.3827) (-3.8254, -7.4159) (-3.8308, -7.4492) (-3.8358, -7.4828) (-3.8403, -7.5165) (-3.8446, -7.5503) (-3.8484, -7.5843) (-3.852, -7.6183) (-3.8552, -7.6525) (-3.858, -7.6868) (-3.8605, -7.7213) (-3.8625, -7.7558) (-3.8643, -7.7905) (-3.8656, -7.8254) (-3.8667, -7.8603) (-3.8674, -7.8953) (-3.8678, -7.9304) (-3.8678, -7.9656) (-3.8676, -8.0009) (-3.8671, -8.0362) (-3.8662, -8.0717) (-3.865, -8.1073) (-3.8635, -8.1429) (-3.8617, -8.1786) (-3.8596, -8.2144) (-3.8572, -8.2502) (-3.8545, -8.2862) (-3.8515, -8.3222) (-3.8482, -8.3582) (-3.8446, -8.3943) (-3.8407, -8.4305) (-3.8366, -8.4668) (-3.8321, -8.5031) (-3.8274, -8.5394) (-3.8224, -8.5758) (-3.8171, -8.6123) (-3.8115, -8.6488) (-3.8057, -8.6853) (-3.7996, -8.7219) (-3.7932, -8.7586) (-3.7865, -8.7952) (-3.7795, -8.832) (-3.7723, -8.8687) (-3.7648, -8.9055) (-3.757, -8.9423) (-3.749, -8.9792) (-3.7407, -9.016) (-3.7322, -9.0529) (-3.7233, -9.0899) (-3.7142, -9.1268) (-3.7049, -9.1638) (-3.6953, -9.2008) (-3.6854, -9.2379) (-3.6752, -9.2749) (-3.6648, -9.312) (-3.6542, -9.349) (-3.6433, -9.3861) (-3.6321, -9.4232) (-3.6229, -9.4529) (-3.616, -9.4752) (-3.6113, -9.49) (-3.6089, -9.4974) knots 0 0 0 0 0 0 0.01428571 0.02857143 0.04285714 0.05714286 0.07142857 0.08571429 0.1 0.11428571 0.12857143 0.14285714 0.15714286 0.17142857 0.18571429 0.2 0.21428571 0.22857143 0.24285714 0.25714286 0.27142857 0.28571429 0.3 0.31428571 0.32857143 0.34285714 0.35714286 0.37142857 0.38571429 0.4 0.41428571 0.42857143 0.44285714 0.45714286 0.47142857 0.48571429 0.5 0.51428571 0.52857143 0.54285714 0.55714286 0.57142857 0.58571429 0.6 0.61428571 0.62857143 0.64285714 0.65714286 0.67142857 0.68571429 0.7 0.71428571 0.72857143 0.74285714 0.75714286 0.77142857 0.78571429 0.8 0.81428571 0.82857143 0.84285714 0.85714286 0.87142857 0.88571429 0.9 0.91428571 0.92857143 0.94285714 0.95714286 0.97142857 0.98571429 1 1 1 1 1 1
  arc A30 (-3.6089, -9.4974) -> (-2.6628, -9.8049) centre (0, 0) ccw
  spline S15 degree 5 poles (-2.6628, -9.8049) (-2.6565, -9.8002) (-2.644, -9.791) (-2.6253, -9.7771) (-2.6004, -9.7584) (-2.5696, -9.735) (-2.5389, -9.7114) (-2.5085, -9.6877) (-2.4783, -9.6638) (-2.4483, -9.6398) (-2.4186, -9.6156) (-2.3891, -9.5914) (-2.3598, -9.5669) (-2.3307, -9.5424) (-2.3018, -9.5177) (-2.2732, -9.4929) (-2.2448, -9.4679) (-2.2166, -9.4428) (-2.1887, -9.4176) (-2.161, -9.3922) (-2.1336, -9.3667) (-2.1064, -9.3411) (-2.0794, -9.3154) (-2.0527, -9.2895) (-2.0262, -9.2635) (-2, -9.2374) (-1.9741, -9.2111) (-1.9484, -9.1847) (-1.9229, -9.1582) (-1.8977, -9.1316) (-1.8728, -9.1049) (-1.8481, -9.078) (-1.8237, -9.051) (-1.7996, -9.0239) (-1.7757, -8.9966) (-1.7522, -8.9693) (-1.7289, -8.9418) (-1.7058, -8.9142) (-1.6831, -8.8865) (-1.6606, -8.8586) (-1.6385, -8.8307) (-1.6166, -8.8026) (-1.5951, -8.7745) (-1.5738, -8.7462) (-1.5529, -8.7178) (-1.5323, -8.6892) (-1.512, -8.6606) (-1.492, -8.6319) (-1.4723, -8.603) (-1.4529, -8.574) (-1.4339, -8.545) (-1.4153, -8.5158) (-1.397, -8.4865) (-1.3791, -8.457) (-1.3616, -8.4275) (-1.3445, -8.3978) (-1.3276, -8.3681) (-1.3112, -8.3383) (-1.2951, -8.3083) (-1.2793, -8.2783) (-1.2641, -8.2481) (-1.2494, -8.2178) (-1.2353, -8.1873) (-1.2219, -8.1567) (-1.2089, -8.126) (-1.1964, -8.0952) (-1.1842, -8.0643) (-1.1722, -8.0334) (-1.1607, -8.0024) (-1.15, -7.9712) (-1.1404, -7.9398) (-1.1342, -7.9144) (-1.1304, -7.8952) (-1.1283, -7.8823) (-1.1273, -7.8758) knots -1 -1 -1 -1 -1 -1 -0.98571429 -0.97142857 -0.95714286 -0.94285714 -0.92857143 -0.91428571 -0.9 -0.88571429 -0.87142857 -0.85714286 -0.84285714 -0.82857143 -0.81428571 -0.8 -0.78571429 -0.77142857 -0.75714286 -0.74285714 -0.72857143 -0.71428571 -0.7 -0.68571429 -0.67142857 -0.65714286 -0.64285714 -0.62857143 -0.61428571 -0.6 -0.58571429 -0.57142857 -0.55714286 -0.54285714 -0.52857143 -0.51428571 -0.5 -0.48571429 -0.47142857 -0.45714286 -0.44285714 -0.42857143 -0.41428571 -0.4 -0.38571429 -0.37142857 -0.35714286 -0.34285714 -0.32857143 -0.31428571 -0.3 -0.28571429 -0.27142857 -0.25714286 -0.24285714 -0.22857143 -0.21428571 -0.2 -0.18571429 -0.17142857 -0.15714286 -0.14285714 -0.12857143 -0.11428571 -0.1 -0.08571429 -0.07142857 -0.05714286 -0.04285714 -0.02857143 -0.01428571 0 0 0 0 0 0
  line L15 (-1.1273, -7.8758) -> (-0.9384, -6.566)
  arc A31 (-0.6607, -6.3496) -> (-0.9384, -6.566) centre (-0.687, -6.6022) ccw
  arc A32 (-0.6607, -6.3496) -> (0.6607, -6.3496) centre (0, 0) ccw
  arc A33 (0.9384, -6.566) -> (0.6607, -6.3496) centre (0.687, -6.6022) ccw
  line L16 (0.9384, -6.566) -> (1.1273, -7.8758)
  spline S16 degree 5 poles (1.1273, -7.8758) (1.1283, -7.8823) (1.1304, -7.8952) (1.1342, -7.9144) (1.1404, -7.9398) (1.15, -7.9712) (1.1607, -8.0024) (1.1722, -8.0334) (1.1842, -8.0643) (1.1964, -8.0952) (1.2089, -8.126) (1.2219, -8.1567) (1.2353, -8.1873) (1.2494, -8.2178) (1.2641, -8.2481) (1.2793, -8.2783) (1.2951, -8.3083) (1.3112, -8.3383) (1.3276, -8.3681) (1.3445, -8.3978) (1.3616, -8.4275) (1.3791, -8.457) (1.397, -8.4865) (1.4153, -8.5158) (1.4339, -8.545) (1.4529, -8.574) (1.4723, -8.603) (1.492, -8.6319) (1.512, -8.6606) (1.5323, -8.6892) (1.5529, -8.7178) (1.5738, -8.7462) (1.5951, -8.7745) (1.6166, -8.8026) (1.6385, -8.8307) (1.6606, -8.8586) (1.6831, -8.8865) (1.7058, -8.9142) (1.7289, -8.9418) (1.7522, -8.9693) (1.7757, -8.9966) (1.7996, -9.0239) (1.8237, -9.051) (1.8481, -9.078) (1.8728, -9.1049) (1.8977, -9.1316) (1.9229, -9.1582) (1.9484, -9.1847) (1.9741, -9.2111) (2, -9.2374) (2.0262, -9.2635) (2.0527, -9.2895) (2.0794, -9.3154) (2.1064, -9.3411) (2.1336, -9.3667) (2.161, -9.3922) (2.1887, -9.4176) (2.2166, -9.4428) (2.2448, -9.4679) (2.2732, -9.4929) (2.3018, -9.5177) (2.3307, -9.5424) (2.3598, -9.5669) (2.3891, -9.5914) (2.4186, -9.6156) (2.4483, -9.6398) (2.4783, -9.6638) (2.5085, -9.6877) (2.5389, -9.7114) (2.5696, -9.735) (2.6004, -9.7584) (2.6253, -9.7771) (2.644, -9.791) (2.6565, -9.8002) (2.6628, -9.8049) knots 0 0 0 0 0 0 0.01428571 0.02857143 0.04285714 0.05714286 0.07142857 0.08571429 0.1 0.11428571 0.12857143 0.14285714 0.15714286 0.17142857 0.18571429 0.2 0.21428571 0.22857143 0.24285714 0.25714286 0.27142857 0.28571429 0.3 0.31428571 0.32857143 0.34285714 0.35714286 0.37142857 0.38571429 0.4 0.41428571 0.42857143 0.44285714 0.45714286 0.47142857 0.48571429 0.5 0.51428571 0.52857143 0.54285714 0.55714286 0.57142857 0.58571429 0.6 0.61428571 0.62857143 0.64285714 0.65714286 0.67142857 0.68571429 0.7 0.71428571 0.72857143 0.74285714 0.75714286 0.77142857 0.78571429 0.8 0.81428571 0.82857143 0.84285714 0.85714286 0.87142857 0.88571429 0.9 0.91428571 0.92857143 0.94285714 0.95714286 0.97142857 0.98571429 1 1 1 1 1 1
  arc A34 (2.6628, -9.8049) -> (3.6089, -9.4974) centre (0, 0) ccw
  spline S17 degree 5 poles (3.6089, -9.4974) (3.6113, -9.49) (3.616, -9.4752) (3.6229, -9.4529) (3.6321, -9.4232) (3.6433, -9.3861) (3.6542, -9.349) (3.6648, -9.312) (3.6752, -9.2749) (3.6854, -9.2379) (3.6953, -9.2008) (3.7049, -9.1638) (3.7142, -9.1268) (3.7233, -9.0899) (3.7322, -9.0529) (3.7407, -9.016) (3.749, -8.9792) (3.757, -8.9423) (3.7648, -8.9055) (3.7723, -8.8687) (3.7795, -8.832) (3.7865, -8.7952) (3.7932, -8.7586) (3.7996, -8.7219) (3.8057, -8.6853) (3.8115, -8.6488) (3.8171, -8.6123) (3.8224, -8.5758) (3.8274, -8.5394) (3.8321, -8.5031) (3.8366, -8.4668) (3.8407, -8.4305) (3.8446, -8.3943) (3.8482, -8.3582) (3.8515, -8.3222) (3.8545, -8.2862) (3.8572, -8.2502) (3.8596, -8.2144) (3.8617, -8.1786) (3.8635, -8.1429) (3.865, -8.1073) (3.8662, -8.0717) (3.8671, -8.0362) (3.8676, -8.0009) (3.8678, -7.9656) (3.8678, -7.9304) (3.8674, -7.8953) (3.8667, -7.8603) (3.8656, -7.8254) (3.8643, -7.7905) (3.8625, -7.7558) (3.8605, -7.7213) (3.858, -7.6868) (3.8552, -7.6525) (3.852, -7.6183) (3.8484, -7.5843) (3.8446, -7.5503) (3.8403, -7.5165) (3.8358, -7.4828) (3.8308, -7.4492) (3.8254, -7.4159) (3.8195, -7.3827) (3.813, -7.3498) (3.8059, -7.3171) (3.7983, -7.2847) (3.7903, -7.2524) (3.7821, -7.2202) (3.7735, -7.1881) (3.7646, -7.1563) (3.755, -7.1248) (3.7443, -7.0938) (3.7344, -7.0696) (3.7262, -7.0518) (3.7203, -7.0401) (3.7172, -7.0343) knots -1 -1 -1 -1 -1 -1 -0.98571429 -0.97142857 -0.95714286 -0.94285714 -0.92857143 -0.91428571 -0.9 -0.88571429 -0.87142857 -0.85714286 -0.84285714 -0.82857143 -0.81428571 -0.8 -0.78571429 -0.77142857 -0.75714286 -0.74285714 -0.72857143 -0.71428571 -0.7 -0.68571429 -0.67142857 -0.65714286 -0.64285714 -0.62857143 -0.61428571 -0.6 -0.58571429 -0.57142857 -0.55714286 -0.54285714 -0.52857143 -0.51428571 -0.5 -0.48571429 -0.47142857 -0.45714286 -0.44285714 -0.42857143 -0.41428571 -0.4 -0.38571429 -0.37142857 -0.35714286 -0.34285714 -0.32857143 -0.31428571 -0.3 -0.28571429 -0.27142857 -0.25714286 -0.24285714 -0.22857143 -0.21428571 -0.2 -0.18571429 -0.17142857 -0.15714286 -0.14285714 -0.12857143 -0.11428571 -0.1 -0.08571429 -0.07142857 -0.05714286 -0.04285714 -0.02857143 -0.01428571 0 0 0 0 0 0
  line L17 (3.7172, -7.0343) -> (3.1002, -5.8636)
  arc A35 (3.1976, -5.5253) -> (3.1002, -5.8636) centre (3.3249, -5.7451) ccw
  arc A36 (3.1976, -5.5253) -> (4.2667, -4.7485) centre (0, 0) ccw
  arc A37 (4.6186, -4.7604) -> (4.2667, -4.7485) centre (4.4365, -4.9375) ccw
  line L18 (4.6186, -4.7604) -> (5.5413, -5.709)
  spline S18 degree 5 poles (5.5413, -5.709) (5.5459, -5.7137) (5.5552, -5.7229) (5.5695, -5.7363) (5.5895, -5.7531) (5.6157, -5.7729) (5.6427, -5.7918) (5.6702, -5.8101) (5.6981, -5.8281) (5.7261, -5.8459) (5.7544, -5.8635) (5.7829, -5.8807) (5.8118, -5.8976) (5.8411, -5.9139) (5.8708, -5.9298) (5.9009, -5.9453) (5.9312, -5.9604) (5.9619, -5.9751) (5.9927, -5.9896) (6.0238, -6.0037) (6.0551, -6.0176) (6.0866, -6.0313) (6.1184, -6.0445) (6.1504, -6.0575) (6.1827, -6.0702) (6.2151, -6.0825) (6.2478, -6.0946) (6.2807, -6.1064) (6.3138, -6.1179) (6.347, -6.1291) (6.3805, -6.14) (6.4141, -6.1507) (6.4479, -6.1611) (6.4819, -6.1713) (6.5161, -6.1811) (6.5505, -6.1907) (6.585, -6.2) (6.6197, -6.2091) (6.6545, -6.2179) (6.6895, -6.2264) (6.7247, -6.2347) (6.76, -6.2427) (6.7954, -6.2504) (6.8311, -6.2579) (6.8668, -6.2652) (6.9027, -6.2722) (6.9387, -6.2789) (6.9749, -6.2854) (7.0112, -6.2916) (7.0477, -6.2976) (7.0842, -6.3033) (7.1209, -6.3088) (7.1577, -6.314) (7.1947, -6.319) (7.2317, -6.3238) (7.2689, -6.3283) (7.3062, -6.3325) (7.3437, -6.3365) (7.3812, -6.3402) (7.4188, -6.3437) (7.4566, -6.347) (7.4944, -6.35) (7.5324, -6.3528) (7.5705, -6.3553) (7.6086, -6.3576) (7.6469, -6.3596) (7.6852, -6.3615) (7.7237, -6.363) (7.7623, -6.3643) (7.8009, -6.3654) (7.8396, -6.3662) (7.8707, -6.3667) (7.894, -6.367) (7.9096, -6.3671) (7.9174, -6.3671) knots 0 0 0 0 0 0 0.01428571 0.02857143 0.04285714 0.05714286 0.07142857 0.08571429 0.1 0.11428571 0.12857143 0.14285714 0.15714286 0.17142857 0.18571429 0.2 0.21428571 0.22857143 0.24285714 0.25714286 0.27142857 0.28571429 0.3 0.31428571 0.32857143 0.34285714 0.35714286 0.37142857 0.38571429 0.4 0.41428571 0.42857143 0.44285714 0.45714286 0.47142857 0.48571429 0.5 0.51428571 0.52857143 0.54285714 0.55714286 0.57142857 0.58571429 0.6 0.61428571 0.62857143 0.64285714 0.65714286 0.67142857 0.68571429 0.7 0.71428571 0.72857143 0.74285714 0.75714286 0.77142857 0.78571429 0.8 0.81428571 0.82857143 0.84285714 0.85714286 0.87142857 0.88571429 0.9 0.91428571 0.92857143 0.94285714 0.95714286 0.97142857 0.98571429 1 1 1 1 1 1
  arc A38 (7.9174, -6.3671) -> (8.5021, -5.5623) centre (0, 0) ccw
  spline S19 degree 5 poles (8.5021, -5.5623) (8.4997, -5.5549) (8.4947, -5.5402) (8.4873, -5.518) (8.4772, -5.4887) (8.4645, -5.4521) (8.4515, -5.4157) (8.4383, -5.3794) (8.425, -5.3433) (8.4114, -5.3074) (8.3976, -5.2716) (8.3837, -5.236) (8.3695, -5.2006) (8.3551, -5.1654) (8.3406, -5.1303) (8.3258, -5.0954) (8.3108, -5.0607) (8.2957, -5.0261) (8.2803, -4.9918) (8.2648, -4.9576) (8.249, -4.9236) (8.233, -4.8899) (8.2169, -4.8563) (8.2005, -4.8229) (8.184, -4.7897) (8.1672, -4.7566) (8.1503, -4.7238) (8.1331, -4.6912) (8.1158, -4.6588) (8.0983, -4.6266) (8.0805, -4.5947) (8.0626, -4.5629) (8.0444, -4.5314) (8.0261, -4.5) (8.0076, -4.4689) (7.9888, -4.4381) (7.9699, -4.4074) (7.9508, -4.377) (7.9314, -4.3468) (7.9119, -4.3168) (7.8922, -4.2871) (7.8722, -4.2577) (7.8521, -4.2285) (7.8318, -4.1995) (7.8112, -4.1708) (7.7904, -4.1424) (7.7695, -4.1142) (7.7483, -4.0863) (7.727, -4.0587) (7.7054, -4.0313) (7.6836, -4.0043) (7.6616, -3.9775) (7.6394, -3.9511) (7.6169, -3.925) (7.5943, -3.8992) (7.5714, -3.8737) (7.5483, -3.8486) (7.525, -3.8237) (7.5015, -3.7991) (7.4778, -3.7748) (7.4538, -3.751) (7.4295, -3.7277) (7.4049, -3.7049) (7.3799, -3.6826) (7.3547, -3.6608) (7.3293, -3.6394) (7.3037, -3.6182) (7.2779, -3.5973) (7.252, -3.5768) (7.2257, -3.5569) (7.1988, -3.5382) (7.1766, -3.5243) (7.1595, -3.5148) (7.1478, -3.5088) (7.142, -3.5059) knots -1 -1 -1 -1 -1 -1 -0.98571429 -0.97142857 -0.95714286 -0.94285714 -0.92857143 -0.91428571 -0.9 -0.88571429 -0.87142857 -0.85714286 -0.84285714 -0.82857143 -0.81428571 -0.8 -0.78571429 -0.77142857 -0.75714286 -0.74285714 -0.72857143 -0.71428571 -0.7 -0.68571429 -0.67142857 -0.65714286 -0.64285714 -0.62857143 -0.61428571 -0.6 -0.58571429 -0.57142857 -0.55714286 -0.54285714 -0.52857143 -0.51428571 -0.5 -0.48571429 -0.47142857 -0.45714286 -0.44285714 -0.42857143 -0.41428571 -0.4 -0.38571429 -0.37142857 -0.35714286 -0.34285714 -0.32857143 -0.31428571 -0.3 -0.28571429 -0.27142857 -0.25714286 -0.24285714 -0.22857143 -0.21428571 -0.2 -0.18571429 -0.17142857 -0.15714286 -0.14285714 -0.12857143 -0.11428571 -0.1 -0.08571429 -0.07142857 -0.05714286 -0.04285714 -0.02857143 -0.01428571 0 0 0 0 0 0
  line L19 (7.142, -3.5059) -> (5.9546, -2.9215)
  arc A39 (5.8346, -2.5905) -> (5.9546, -2.9215) centre (6.0668, -2.6936) ccw
  circle A40 centre (0, 0) radius 3.1115
  circle A41 centre (0, 0) radius 6.3839
  circle A42 centre (0, 0) radius 3.1115
  constraint coincident A0.centre A2.centre
  constraint coincident A15.start A41
sketch "Sketch2" plane through (0, 0, 12.7) normal (0, 0, 1) x (1, 0, 0)
  circle A0 centre (0, 0) radius 3.1115
  circle A1 centre (0, 0) radius 6.3839
  circle A2 centre (0, 0) radius 2.9845
  dimension "d43" = 5.969
  constraint coincident A0.centre A1.centre
  measures "d43" diameter of A2
sketch "Sketch1 (2)" plane through (0, 0, 0) normal (0, 0, 1) x (1, 0, 0) in component "Spur Gear (8 teeth)"
  circle A0 centre (0, 0) radius 3.5052
  circle A1 centre (0, 0) radius 3.175
extrude "Extrude1" add sketch "Sketch1 (2)" along normal blind 7.62 in component "Spur Gear (8 teeth)"